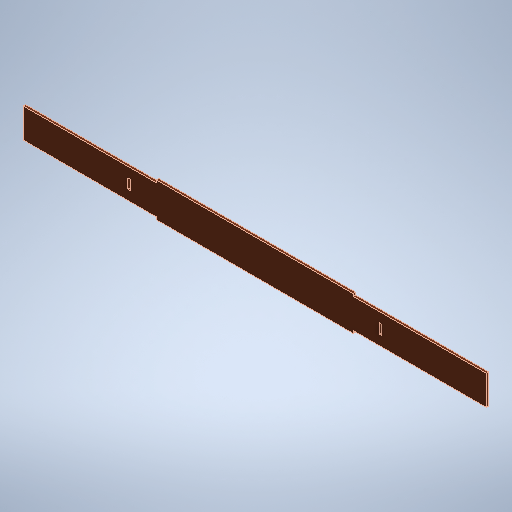
# Autodesk Inventor part: Table-Base Fixation 2nd
Saved by Autodesk Inventor 2025.4 (Build 294407000, 407)
## iProperties
Created: 2026-05-09
Part Number: Table-Base Fixation 2nd
Material: Generic
Document SubType Name: Sheet Metal
Designer: lenovo
Density: 1 g/cm^3
Sheet Metal Rule: Default_mm
Appearance: Default(1)
Author: lenovo
Autodesk Inventor part; units mm, degrees
ref_plane "YZ Plane" through (0, 0, 0) normal (1, 0, 0) x (0, 1, 0)
ref_plane "XZ Plane" through (0, 0, 0) normal (0, 1, 0) x (-1, 0, 0)
ref_plane "XY Plane" through (0, 0, 0) normal (0, 0, 1) x (1, 0, 0)
sketch "Sketch1" plane through (0, 0, 0) normal (0, 0, 1) x (1, 0, 0)
  line L0 (-470, -30) -> (470, -30)
  line L1 (470, -30) -> (470, 30)
  line L2 (470, 30) -> (-470, 30)
  line L3 (-470, 30) -> (-470, -30)
  line L4 (-470, -30) -> (470, 30) construction
  line L5 (470, -30) -> (-470, 30) construction
  line L6 (200, 35) -> (-200, 35)
  line L7 (-200, 35) -> (-200, 30)
  line L8 (-200, 30) -> (200, 30)
  line L9 (200, 30) -> (200, 35)
  line L10 (200, 35) -> (-200, 30) construction
  line L11 (-200, 35) -> (200, 30) construction
  line L12 (-470, 0) -> (470, 0)
  line L13 (200, -35) -> (-200, -35)
  line L14 (-200, -35) -> (-200, -30)
  line L15 (-200, -30) -> (200, -30)
  line L16 (200, -30) -> (200, -35)
  line L17 (200, -35) -> (-200, -30) construction
  line L18 (-200, -35) -> (200, -30) construction
  point P0 (0, 0)
  point P1 (0, 32.5)
  point P2 (0, 30)
  point P3 (0, -32.5)
  point P4 (0, -30)
  dimension "d0" = 940
  dimension "d1" = 60
  dimension "d2" = 400
  dimension "d3" = 5
  measures "d0" distance of L2.end L1.end
  measures "d1" distance of L1.end L0.end
  measures "d2" distance of L8.end L7.end
  measures "d3" distance of L7.end L6.end
extrude "Plate1" add sketch "Sketch1" along normal blind 5
sketch "Sketch2" plane through (0, 0, 5) normal (0, 0, 1) x (1, 0, 0)
  line L0 (-257.54, 10) -> (-252.46, 10)
  line L1 (-252.46, 10) -> (-252.46, -10)
  line L2 (-252.46, -10) -> (-257.54, -10)
  line L3 (-257.54, -10) -> (-257.54, 10)
  line L4 (-257.54, 10) -> (-252.46, -10) construction
  line L5 (-252.46, 10) -> (-257.54, -10) construction
  line L6 (200, 35) -> (-200, 35) projected
  line L7 (0, 35) -> (0, -35)
  line L8 (-200, -35) -> (200, -35) projected
  line L9 (257.54, 10) -> (252.46, 10)
  line L10 (252.46, 10) -> (252.46, -10)
  line L11 (252.46, -10) -> (257.54, -10)
  line L12 (257.54, -10) -> (257.54, 10)
  line L13 (257.54, 10) -> (252.46, -10) construction
  line L14 (252.46, 10) -> (257.54, -10) construction
  point P0 (0, 0)
  point P1 (-255, 0)
  point P2 (255, 0)
  point P3 (0, 0)
  dimension "d5" = 5.08
  dimension "d6" = 20
  dimension "d7" = 510
  constraints: 26 end point, 5 midpoint, 5 symmetric about line, 2 parallel, 1 horizontal, 1 horizontal alignment, 1 perpendicular
  measures "d5" distance of L0.start L0.end
  measures "d6" distance between parallel lines of L0 L2
  measures "d7" diameter of point (-255, 0) L7
extrude "Cut1" cut sketch "Sketch2" against normal blind 5
equation "\"d8\" = Thickness"
equation "\"d4\" = Thickness"
equation "\"BendRadius\" = Thickness"
equation "\"BendReliefWidth\" = Thickness"
equation "\"BendReliefDepth\" = 0.5 * Thickness"
equation "\"TransitionRadius\" = BendRadius"
equation "\"JacobiRadiusSize\" = BendRadius"
equation "\"GapSize\" = Thickness"
equation "\"Thickness\" = 5"
body "Solid1"
